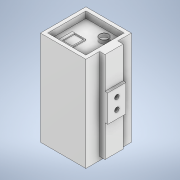
# Autodesk Inventor part: camera
Saved by Autodesk Inventor 2021.2 (Build 252289000, 289)
## iProperties
Created: 2021-02-17
Part Number: camera
Material: PAEK Plastic
Document SubType Name: Modeling
Designer: yxion
Density: 1.32 g/cm^3
Appearance: Smooth - White
Author: yxion
Autodesk Inventor part; units mm, degrees
ref_plane "YZ Plane" through (0, 0, 0) normal (1, 0, 0) x (0, 1, 0)
ref_plane "XZ Plane" through (0, 0, 0) normal (0, 1, 0) x (-1, 0, 0)
ref_plane "XY Plane" through (0, 0, 0) normal (0, 0, 1) x (1, 0, 0)
sketch "Sketch1" plane through (0, 0, 0) normal (0, 1, 0) x (-1, 0, 0)
  line L0 (5.8173, 9.2628) -> (2.8173, 9.2628)
  line L1 (2.8173, 9.2628) -> (2.8173, -10.7372)
  line L2 (2.8173, -10.7372) -> (5.8173, -10.7372)
  line L3 (5.8173, -10.7372) -> (5.8173, 9.2628)
  point P0 (0, 0)
  dimension "d0" = 20
  dimension "d1" = 3
  constraints: 8 end point, 2 parallel, 1 horizontal, 1 perpendicular
  measures "d0" distance of L2.end L0.start
  measures "d1" distance of L1.end L2.end
extrude "Extrusion1" add sketch "Sketch1" along normal blind 30
sketch "Sketch2" plane through (-2.8173, 0, 9.2628) normal (1, 0, 0) x (0, 0, -1)
  circle A0 centre (10, 21) radius 2.5
  circle A1 centre (10, 9) radius 2.5
  line L0 (0, 30) -> (20, 30) projected
  line L1 (0, 0) -> (20, 0) projected
  line L2 (10, 30) -> (10, 21) construction
  line L3 (10, 9) -> (10, 0) construction
  point P0 (9.2628, 0)
  dimension "d4" = 5
  dimension "d5" = 5
  dimension "d41" = 12
  constraints: 4 end point, 2 centre point, 2 midpoint, 1 collinear, 1 vertical
  measures "d4" diameter of A0
  measures "d5" diameter of A1
  measures "d41" distance of L3.start L2.end
sketch "Sketch3" plane through (-5.8173, 0, -10.7372) normal (-1, 0, 0) x (0, 0, 1)
  line L0 (0, 65) -> (20, 65)
  line L1 (20, 65) -> (20, -35)
  line L2 (20, -35) -> (0, -35)
  line L3 (0, -35) -> (0, 65)
  line L4 (20, 0) -> (20, 30) projected
  line L5 (0, 0) -> (0, 30) projected
  line L6 (0, 30) -> (20, 30) projected
  line L7 (0, 0) -> (20, 0) projected
  point P0 (10.7372, 0)
  dimension "d9" = 35
  dimension "d10" = 35
  constraints: 8 end point, 2 collinear, 2 parallel, 1 horizontal, 1 perpendicular
  measures "d9" distance between parallel lines of L0 L6
  measures "d10" distance between parallel lines of L2 L7
extrude "Extrusion2" add sketch "Sketch3" along normal blind 6
sketch "Sketch4" plane through (-5.8173, 65, 9.2628) normal (0, 1, 0) x (1, 0, 0)
  line L0 (-56, 35) -> (-6, 35)
  line L1 (-6, 35) -> (-6, -15)
  line L2 (-6, -15) -> (-56, -15)
  line L3 (-56, -15) -> (-56, 35)
  line L4 (-6, 0) -> (-6, 20) projected
  line L5 (0, 20) -> (-6, 20) projected
  line L6 (-6, 10) -> (-56, 10) construction
  line L7 (-31, 35) -> (-31, 10) construction
  line L8 (-31, -15) -> (-31, 10) construction
  line L9 (-10, 31) -> (-52, 31)
  line L10 (-52, 31) -> (-52, -11)
  line L11 (-52, -11) -> (-10, -11)
  line L12 (-10, -11) -> (-10, 31)
  point P0 (5.8173, 9.2628)
  dimension "d13" = 50
  dimension "d14" = 50
  dimension "d16" = 4
  constraints: 22 end point, 5 equal length, 5 midpoint, 3 perpendicular, 2 collinear, 1 horizontal, 3 other
  measures "d13" distance of L0.start L0.end
  measures "d14" distance of L2.end L0.start
  measures "d16" distance between parallel lines of L9 L0
extrude "Extrusion3" add sketch "Sketch4" against normal blind 7
sketch "Sketch5" plane through (-5.8173, 58, 9.2628) normal (0, -1, 0) x (1, 0, 0)
  line L0 (-56, 15) -> (-56, -35) projected
  line L1 (-56, -35) -> (-6, -35) projected
  line L2 (-6, -35) -> (-6, -20) projected
  line L3 (-6, 0) -> (-6, -20) projected
  line L4 (-6, 0) -> (-6, 15) projected
  line L5 (-6, 15) -> (-56, 15) projected
  line L6 (-10, 11) -> (-10, -31) projected
  line L7 (-10, -31) -> (-52, -31) projected
  line L8 (-52, -31) -> (-52, 11) projected
  line L9 (-52, 11) -> (-10, 11) projected
  point P0 (5.8173, -9.2628)
extrude "Extrusion4" add sketch "Sketch5" along normal blind 90 contours L5 L4 L3 L2 L1 L0 | L6 L7 L8 L9
sketch "Sketch6" plane through (-5.8173, -32, 9.2628) normal (0, -1, 0) x (1, 0, 0)
  line L0 (-10, 11) -> (-10, -31) projected
  line L1 (-52, 11) -> (-10, 11) projected
  line L2 (-52, -31) -> (-52, 11) projected
  line L3 (-10, -31) -> (-52, -31) projected
  line L4 (-6, 15) -> (-56, 15) projected
  line L5 (-56, 15) -> (-56, -35) projected
  line L6 (-56, -35) -> (-6, -35) projected
  line L7 (-6, -35) -> (-6, -20) projected
  line L8 (-6, 0) -> (-6, -20) projected
  line L9 (-6, 0) -> (-6, 15) projected
  point P0 (5.8173, -9.2628)
extrude "Extrusion5" add sketch "Sketch6" along normal blind 7
extrude "Extrusion6" cut sketch "Sketch2" against normal blind 7
sketch "Sketch7" plane through (-5.8173, -32, 9.2628) normal (0, -1, 0) x (1, 0, 0)
  circle A0 centre (-31.392, -9.2628) radius 20
  line L0 (-10, 11) -> (-52, 11) projected
  line L1 (-52, 11) -> (-52, -31) projected
  line L2 (-52, -31) -> (-10, -31) projected
  line L3 (-10, -31) -> (-10, 11) projected
  line L4 (-6, 15) -> (-56, 15) projected
  line L5 (-56, 15) -> (-56, -35) projected
  line L6 (-56, -35) -> (-6, -35) projected
  line L7 (-6, -35) -> (-6, 15) projected
  line L8 (-10, 11) -> (-10, -31) projected
  line L9 (-10, -31) -> (-52, -31) projected
  line L10 (-52, -31) -> (-52, 11) projected
  line L11 (-52, 11) -> (-10, 11) projected
  point P0 (5.8173, -9.2628)
  dimension "d25" = 40
  constraints: 1 centre point
  measures "d25" diameter of A0
extrude "Extrusion7" add sketch "Sketch7" along normal blind 7 contours L3 L2 L1 L0
sketch "Sketch8" plane through (-5.8173, 58, 9.2628) normal (0, 1, 0) x (1, 0, 0)
  circle A0 centre (-21, 20) radius 5
  line L0 (-46, -5) -> (-31, -5)
  line L1 (-31, -5) -> (-31, 10)
  line L2 (-31, 10) -> (-46, 10)
  line L3 (-46, 10) -> (-46, -5)
  line L4 (-6, 35) -> (-56, 35) projected
  line L5 (-6, 20) -> (-6, 35) projected
  line L6 (-56, -15) -> (-6, -15) projected
  line L7 (-56, 35) -> (-56, -15) projected
  circle A1 centre (-21, 20) radius 4.5053
  line L8 (-42.9073, -3.8349) -> (-32.3073, -3.8349)
  line L9 (-32.3073, -3.8349) -> (-32.3073, 9.1651)
  line L10 (-32.3073, 9.1651) -> (-42.9073, 9.1651)
  line L11 (-42.9073, 9.1651) -> (-42.9073, -3.8349)
  point P0 (5.8173, 9.2628)
  dimension "d28" = 15
  dimension "d29" = 15
  dimension "d30" = 10
  dimension "d31" = 15
  dimension "d32" = 15
  dimension "d33" = 10
  dimension "d34" = 10
  dimension "d35" = 10.6
  dimension "d36" = 13
  constraints: 16 end point, 4 parallel, 2 centre point, 2 horizontal, 2 perpendicular
  measures "d28" distance of L2.end L0.start
  measures "d29" distance of L1.end L2.end
  measures "d30" diameter of A0
  measures "d31" distance from line of L4 A0.centre
  measures "d32" distance from line of L5 A0.centre
  measures "d33" distance between parallel lines of L6 L0
  measures "d34" distance between parallel lines of L7 L3
  measures "d35" distance of L9.end L10.end
  measures "d36" distance of L10.end L8.start
extrude "Extrusion8" add sketch "Sketch8" along normal blind 1
sketch "Sketch10" plane through (-26.8173, 59, -10.7372) normal (0, 1, 0) x (1, 0, 0)
  circle A0 centre (0, 0) radius 4.5053 projected
  circle A1 centre (0, 0) radius 5 projected
  point P0 (26.8173, -10.7372)
extrude "Extrusion9" add sketch "Sketch10" along normal blind 2.5875
body "Solid1"
